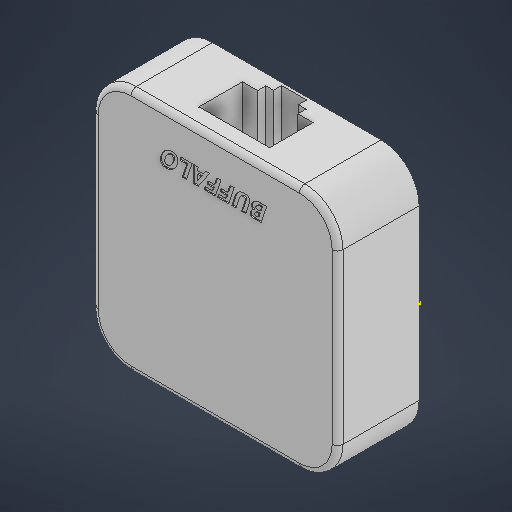
# Autodesk Inventor part: WMR-433-BK
Saved by Autodesk Inventor 2026.1 (Build 301233020, 233B)
## iProperties
Created: 2026-03-19
Part Number: WMR-433-BK
Material: 一般
Document SubType Name: Modeling
Designer: kamada
Density: 1 g/cm^3
Appearance: 既定
Author: kamada
Autodesk Inventor part; units mm, degrees
ref_plane "YZ Plane" through (0, 0, 0) normal (1, 0, 0) x (0, 1, 0)
ref_plane "XZ Plane" through (0, 0, 0) normal (0, 1, 0) x (-1, 0, 0)
ref_plane "XY Plane" through (0, 0, 0) normal (0, 0, 1) x (1, 0, 0)
sketch "スケッチ1" plane through (0, 0, 0) normal (0, 0, 1) x (1, 0, 0)
  line L0 (-22.5, 22.5) -> (22.5, 22.5)
  line L1 (22.5, 22.5) -> (22.5, -22.5)
  line L2 (22.5, -22.5) -> (-22.5, -22.5)
  line L3 (-22.5, -22.5) -> (-22.5, 22.5)
  point P0 (0, 0)
  point P1 (0, 22.5)
  point P2 (22.5, 0)
  dimension "d0" = 45
  dimension "d1" = 45
  constraints: 8 end point, 2 midpoint, 2 parallel, 1 horizontal, 1 horizontal alignment, 1 perpendicular, 1 vertical alignment
  measures "d0" distance of L0.end L1.end
  measures "d1" distance of L0.start L0.end
extrude "押し出し1" add sketch "スケッチ1" along normal blind 15
sketch "スケッチ2" plane through (-22.5, 22.5, 0) normal (0, 1, 0) x (1, 0, 0)
  line L0 (30.5, -13.8) -> (14.5, -13.8)
  line L1 (14.5, -13.8) -> (14.5, 0)
  line L2 (14.5, 0) -> (30.5, 0)
  line L3 (30.5, 0) -> (30.5, -13.8)
  line L4 (45, 0) -> (0, 0) projected
  line L5 (0, 0) -> (0, -15) projected
  line L6 (45, -15) -> (0, -15) projected
  line L7 (45, 0) -> (45, -15) projected
  line L8 (29, -11.5) -> (16, -11.5)
  line L9 (16, -11.5) -> (16, -3.5)
  line L10 (16, -3.5) -> (29, -3.5)
  line L11 (29, -3.5) -> (29, -11.5)
  line L12 (24.8, -2) -> (20.2, -2)
  line L13 (20.2, -2) -> (20.2, -0.5)
  line L14 (20.2, -0.5) -> (24.8, -0.5)
  line L15 (24.8, -0.5) -> (24.8, -2)
  line L16 (26.2, -3.5) -> (18.8, -3.5)
  line L17 (18.8, -3.5) -> (18.8, -2)
  line L18 (18.8, -2) -> (26.2, -2)
  line L19 (26.2, -2) -> (26.2, -3.5)
  point P0 (22.5, 0)
  point P1 (22.5, -13.8)
  point P2 (22.5, -15)
  point P3 (22.5, 0)
  point P4 (22.5, -2)
  point P5 (22.5, -2)
  point P6 (22.5, -3.5)
  point P7 (22.5, -3.5)
  point P8 (22.5, -0.5)
  dimension "d4" = 16
  dimension "d5" = 13.8
  dimension "d6" = 13
  dimension "d7" = 8
  dimension "d8" = 4.6
  dimension "d9" = 7.4
  dimension "d10" = 1.5
  dimension "d11" = 1.5
  dimension "d12" = 0.5
  constraints: 32 end point, 10 midpoint, 8 parallel, 4 horizontal, 4 perpendicular, 2 coincident, 2 vertical alignment, 1 horizontal alignment
  measures "d4" distance of L1.end L2.end
  measures "d5" distance of L0.end L1.end
  measures "d6" distance of L9.end L10.end
  measures "d7" distance of L8.end L9.end
  measures "d8" distance of L13.end L14.end
  measures "d9" distance of L17.end L18.end
  measures "d10" distance of L12.end L13.end
  measures "d11" distance of L16.end L17.end
  measures "d12" distance between parallel lines of L14 L2
extrude "押し出し2" cut sketch "スケッチ2" against normal blind 10 contours L8 L9 L10 L11 | L10 L17 L18 L12 L19 | L12 L13 L14 L15
fillet "フィレット1" radius 7 4 edges at (22.5, 22.5, 7.5) (-22.5, 22.5, 7.5) (-22.5, -22.5, 7.5) (22.5, -22.5, 7.5)
fillet "フィレット2" radius 1 8 edges at (-20.4497, 20.4497, 15) (-22.5, 0, 15) (-20.4497, -20.4497, 15) (0, -22.5, 15) (20.4497, -20.4497, 15) (22.5, 0, 15) (20.4497, 20.4497, 15) (0, 22.5, 15)
sketch "スケッチ3" plane through (22.5, -15.5, 0) normal (1, 0, 0) x (0, 0, -1)
  point P0 (0, 15.5)
sketch "スケッチ4" plane through (0, 0, 15) normal (0, 0, 1) x (1, 0, 0)
  line L0 (9.7877, 13.2402) -> (-9.7877, 13.2402) construction
  line L1 (-9.7877, 13.2402) -> (-9.7877, 17.0239) construction
  line L2 (-9.7877, 17.0239) -> (9.7877, 17.0239) construction
  line L3 (9.7877, 17.0239) -> (9.7877, 13.2402) construction
  line L4 (-15.5, 21.5) -> (15.5, 21.5) projected
  spline S0 degree 2 poles (6.7154, 15.4201) (6.7945, 15.6475) (7.0837, 15.9911) (7.2666, 16.1048) knots 0 0 0 1 2 2 2
  spline S1 degree 2 poles (7.2666, 16.1048) (7.4841, 16.2407) (7.934, 16.3544) (8.2528, 16.3544) knots 0 0 0 1 2 2 2
  line L5 (8.2528, 16.3544) -> (9.4713, 16.3544)
  line L6 (9.4713, 16.3544) -> (8.4357, 13.3044)
  line L7 (8.4357, 13.3044) -> (7.3581, 13.3044)
  spline S2 degree 2 poles (7.3581, 13.3044) (7.0219, 13.3044) (6.6957, 13.3563) (6.5721, 13.4379) knots 0 0 0 1 2 2 2
  spline S3 degree 2 poles (6.5721, 13.4379) (6.4361, 13.5244) (6.3768, 13.821) (6.4411, 14.0138) knots 0 0 0 1 2 2 2
  spline S4 degree 2 poles (6.4411, 14.0138) (6.5177, 14.2362) (6.8588, 14.5847) (7.0812, 14.6663) knots 0 0 0 1 2 2 2
  line L8 (7.0812, 14.6663) -> (7.0887, 14.6811)
  spline S5 degree 2 poles (7.0887, 14.6811) (6.8267, 14.7404) (6.6116, 15.1087) (6.7154, 15.4201) knots 0 0 0 1 2 2 2
  spline S6 degree 2 poles (7.5039, 15.4078) (7.4545, 15.2644) (7.5138, 15.1038) (7.6151, 15.0618) knots 0 0 0 1 2 2 2
  spline S7 degree 2 poles (7.6151, 15.0618) (7.6744, 15.0346) (7.9142, 15.0296) (8.1193, 15.0296) knots 0 0 0 1 2 2 2
  line L9 (8.1193, 15.0296) -> (8.2602, 15.0296)
  line L10 (8.2602, 15.0296) -> (8.5222, 15.7983)
  line L11 (8.5222, 15.7983) -> (8.4802, 15.7983)
  spline S8 degree 2 poles (8.4802, 15.7983) (8.1836, 15.7983) (7.9513, 15.7909) (7.8153, 15.739) knots 0 0 0 1 2 2 2
  spline S9 degree 2 poles (7.8153, 15.739) (7.6967, 15.692) (7.541, 15.519) (7.5039, 15.4078) knots 0 0 0 1 2 2 2
  spline S10 degree 2 poles (7.2716, 14.1645) (7.2468, 14.0904) (7.2691, 13.9347) (7.3358, 13.9001) knots 0 0 0 1 2 2 2
  spline S11 degree 2 poles (7.3358, 13.9001) (7.4001, 13.8655) (7.6052, 13.8605) (7.8104, 13.8605) knots 0 0 0 1 2 2 2
  line L12 (7.8104, 13.8605) -> (7.8623, 13.8605)
  line L13 (7.8623, 13.8605) -> (8.0823, 14.5081)
  line L14 (8.0823, 14.5081) -> (7.9859, 14.5081)
  spline S12 degree 2 poles (7.9859, 14.5081) (7.7906, 14.5081) (7.6299, 14.5007) (7.5335, 14.4611) knots 0 0 0 1 2 2 2
  spline S13 degree 2 poles (7.5335, 14.4611) (7.4273, 14.4167) (7.3062, 14.2659) (7.2716, 14.1645) knots 0 0 0 1 2 2 2
  spline S14 degree 2 poles (5.3832, 16.4187) (5.9987, 16.4187) (6.4584, 15.8255) (6.2656, 15.2521) knots 0 0 0 1 2 2 2
  line L15 (6.2656, 15.2521) -> (5.6032, 13.3044)
  line L16 (5.6032, 13.3044) -> (4.837, 13.3044)
  line L17 (4.837, 13.3044) -> (5.4821, 15.2076)
  spline S15 degree 2 poles (5.4821, 15.2076) (5.5908, 15.5264) (5.4574, 15.8378) (5.1855, 15.8378) knots 0 0 0 1 2 2 2
  spline S16 degree 2 poles (5.1855, 15.8378) (4.921, 15.8378) (4.5725, 15.5388) (4.4588, 15.2076) knots 0 0 0 1 2 2 2
  line L18 (4.4588, 15.2076) -> (3.8137, 13.3044)
  line L19 (3.8137, 13.3044) -> (3.0475, 13.3044)
  line L20 (3.0475, 13.3044) -> (3.7075, 15.2496)
  spline S17 degree 2 poles (3.7075, 15.2496) (3.9002, 15.8131) (4.7505, 16.4187) (5.3832, 16.4187) knots 0 0 0 1 2 2 2
  line L21 (0.613, 13.8853) -> (1.8933, 13.8853)
  line L22 (1.8933, 13.8853) -> (2.091, 14.4611)
  line L23 (2.091, 14.4611) -> (0.912, 14.4611)
  line L24 (0.912, 14.4611) -> (1.1098, 15.042)
  line L25 (1.1098, 15.042) -> (2.2887, 15.042)
  line L26 (2.2887, 15.042) -> (2.7336, 16.3544)
  line L27 (2.7336, 16.3544) -> (3.4949, 16.3544)
  line L28 (3.4949, 16.3544) -> (2.4593, 13.3044)
  line L29 (2.4593, 13.3044) -> (0.4177, 13.3044)
  line L30 (0.4177, 13.3044) -> (0.613, 13.8853)
  line L31 (-1.8241, 13.8853) -> (-0.5438, 13.8853)
  line L32 (-0.5438, 13.8853) -> (-0.346, 14.4611)
  line L33 (-0.346, 14.4611) -> (-1.525, 14.4611)
  line L34 (-1.525, 14.4611) -> (-1.3273, 15.042)
  line L35 (-1.3273, 15.042) -> (-0.1483, 15.042)
  line L36 (-0.1483, 15.042) -> (0.2966, 16.3544)
  line L37 (0.2966, 16.3544) -> (1.0579, 16.3544)
  line L38 (1.0579, 16.3544) -> (0.0222, 13.3044)
  line L39 (0.0222, 13.3044) -> (-2.0193, 13.3044)
  line L40 (-2.0193, 13.3044) -> (-1.8241, 13.8853)
  line L41 (-1.0504, 16.3544) -> (-3.1167, 13.3044)
  line L42 (-3.1167, 13.3044) -> (-3.9521, 13.3044)
  line L43 (-3.9521, 13.3044) -> (-3.9472, 16.3544)
  line L44 (-3.9472, 16.3544) -> (-3.1588, 16.3544)
  line L45 (-3.1588, 16.3544) -> (-3.181, 15.7316)
  line L46 (-3.181, 15.7316) -> (-2.2195, 15.7316)
  line L47 (-2.2195, 15.7316) -> (-1.8167, 16.3544)
  line L48 (-1.8167, 16.3544) -> (-1.0504, 16.3544)
  line L49 (-3.2008, 15.1779) -> (-3.2304, 14.1695)
  line L50 (-3.2304, 14.1695) -> (-2.5754, 15.1779)
  line L51 (-2.5754, 15.1779) -> (-3.2008, 15.1779)
  line L52 (-6.2854, 16.3544) -> (-4.2512, 16.3544)
  line L53 (-4.2512, 16.3544) -> (-5.2868, 13.3044)
  line L54 (-5.2868, 13.3044) -> (-6.053, 13.3044)
  line L55 (-6.053, 13.3044) -> (-5.2152, 15.7736)
  line L56 (-5.2152, 15.7736) -> (-6.4831, 15.7736)
  line L57 (-6.4831, 15.7736) -> (-6.2854, 16.3544)
  spline S18 degree 2 poles (-9.9459, 14.8294) (-9.6938, 15.5709) (-8.6161, 16.4187) (-7.9265, 16.4187) knots 0 0 0 1 2 2 2
  spline S19 degree 2 poles (-7.9265, 16.4187) (-7.237, 16.4187) (-6.7426, 15.561) (-6.9923, 14.8294) knots 0 0 0 1 2 2 2
  spline S20 degree 2 poles (-6.9923, 14.8294) (-7.2419, 14.0953) (-8.3171, 13.2402) (-9.0066, 13.2402) knots 0 0 0 1 2 2 2
  spline S21 degree 2 poles (-9.0066, 13.2402) (-9.6962, 13.2402) (-10.1955, 14.0904) (-9.9459, 14.8294) knots 0 0 0 1 2 2 2
  spline S22 degree 2 poles (-9.1549, 14.8294) (-9.2464, 14.5551) (-9.2662, 14.172) (-9.2118, 14.0509) knots 0 0 0 1 2 2 2
  spline S23 degree 2 poles (-9.2118, 14.0509) (-9.1574, 13.9248) (-8.9473, 13.816) (-8.8139, 13.816) knots 0 0 0 1 2 2 2
  spline S24 degree 2 poles (-8.8139, 13.816) (-8.673, 13.816) (-8.4085, 13.9174) (-8.2602, 14.0459) knots 0 0 0 1 2 2 2
  spline S25 degree 2 poles (-8.2602, 14.0459) (-8.1243, 14.1645) (-7.8746, 14.5575) (-7.7832, 14.8294) knots 0 0 0 1 2 2 2
  spline S26 degree 2 poles (-7.7832, 14.8294) (-7.6868, 15.1112) (-7.672, 15.4819) (-7.7239, 15.608) knots 0 0 0 1 2 2 2
  spline S27 degree 2 poles (-7.7239, 15.608) (-7.7807, 15.734) (-7.9933, 15.8428) (-8.1243, 15.8428) knots 0 0 0 1 2 2 2
  spline S28 degree 2 poles (-8.1243, 15.8428) (-8.2602, 15.8428) (-8.5519, 15.7266) (-8.6878, 15.603) knots 0 0 0 1 2 2 2
  spline S29 degree 2 poles (-8.6878, 15.603) (-8.8312, 15.4696) (-9.0561, 15.1161) (-9.1549, 14.8294) knots 0 0 0 1 2 2 2
  point P0 (0, 0)
  point P1 (0, 13.2402)
  point P2 (0, 21.5)
  dimension "d0" = 45
  dimension "d1" = 45
  constraints: 2 midpoint, 1 vertical alignment, 2 other
extrude "押し出し3" cut sketch "スケッチ4" against normal blind 0.2
sketch "スケッチ5" plane through (-22.5, -15.5, 0) normal (-1, 0, 0) x (0, 0, 1)
  line L0 (7.5905, 10.1152) -> (7.5905, 2.6152)
  line L1 (7.5905, 10.1152) -> (5.0905, 10.1152)
  line L2 (5.0905, 10.1152) -> (5.0905, 2.6152)
  line L3 (5.0905, 2.6152) -> (7.5905, 2.6152)
  line L4 (7.5905, 2.6152) -> (7.5905, 10.1152)
  line L5 (7.5905, 2.6152) -> (6.3405, 2.6152)
  line L6 (6.3405, 2.6152) -> (6.3405, 10.1152)
  line L7 (6.3405, 10.1152) -> (7.5905, 10.1152)
  line L8 (7.5905, 10.1152) -> (7.5905, 2.6152)
  line L9 (6.3405, 10.1152) -> (5.0905, 8.8652)
  line L10 (6.3405, 10.1152) -> (8.1082, 10.1152) construction
  line L11 (6.3405, 2.6152) -> (5.0905, 3.8652)
  line L12 (6.3405, 2.6152) -> (8.1082, 2.6152) construction
  point P0 (0, 15.5)
  dimension "d19" = 7.5
  dimension "d20" = 2.5
  dimension "d21" = 135
  dimension "d22" = 135
  constraints: 26 end point, 4 horizontal, 4 parallel, 2 equal length, 2 perpendicular, 2 point on line, 1 midpoint, 1 vertical
  measures "d19" distance of L0.start L0.end
  measures "d20" distance of L3.end L2.end
  measures "d21" angle of L9 L10
  measures "d22" angle of L12 L11
extrude "押し出し4" cut sketch "スケッチ5" against normal blind 5 contours L0 L3 L6 L1 | L6 L11 L2 L9
equation "\"d1\" = d0"
equation "\"d11\" = d10"
